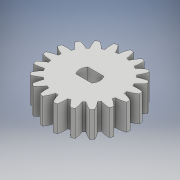
# Autodesk Inventor part: Gear19
Saved by Autodesk Inventor 2018.3 (Build 223284000, 284)
## iProperties
Created: 2019-04-15
Part Number: Gear19
Material: 一般
Document SubType Name: Modeling
Designer: shun2
Density: 1 g/cm^3
Appearance: 既定
Author: shun2
Autodesk Inventor part; units mm, degrees
ref_plane "YZ Plane" through (0, 0, 0) normal (1, 0, 0) x (0, 1, 0)
ref_plane "XZ Plane" through (0, 0, 0) normal (0, 1, 0) x (-1, 0, 0)
ref_plane "XY Plane" through (0, 0, 0) normal (0, 0, 1) x (1, 0, 0)
sketch "スケッチ1" plane through (0, 0, 0) normal (0, 0, 1) x (1, 0, 0)
  arc A0 (-3.8168, 9.7817) -> (-3.6234, 7.4117) centre (4.2362, 9.2462) ccw
  arc A1 (-3.6234, 7.4117) -> (-4.2231, 7.0872) centre (0, 0) ccw
  arc A2 (-4.2231, 7.0872) -> (-6.1013, 8.5454) centre (-10.0576, 1.5108) ccw
  arc A3 (-6.1013, 8.5454) -> (-6.7861, 8.0124) centre (0, 0) ccw
  arc A4 (-6.7861, 8.0124) -> (-5.8336, 5.8336) centre (1.0044, 10.1207) ccw
  arc A5 (-5.8336, 5.8336) -> (-6.2954, 5.332) centre (0, 0) ccw
  arc A6 (-6.2954, 5.332) -> (-8.5454, 6.1013) centre (-10.0032, -1.8368) ccw
  arc A7 (-8.5454, 6.1013) -> (-9.0201, 5.3748) centre (0, 0) ccw
  arc A8 (-9.0201, 5.3748) -> (-7.4117, 3.6234) centre (-2.3362, 9.8985) ccw
  arc A9 (-7.4117, 3.6234) -> (-7.6856, 2.9989) centre (0, 0) ccw
  arc A10 (-7.6856, 2.9989) -> (-10.0635, 2.996) centre (-8.8648, -4.9853) ccw
  arc A11 (-10.0635, 2.996) -> (-10.2765, 2.1548) centre (0, 0) ccw
  arc A12 (-10.2765, 2.1548) -> (-8.1866, 1.0205) centre (-5.4236, 8.6036) ccw
  arc A13 (-8.1866, 1.0205) -> (-8.243, 0.3409) centre (0, 0) ccw
  arc A14 (-8.243, 0.3409) -> (-10.491, -0.4339) centre (-6.7658, -7.5935) ccw
  arc A15 (-10.491, -0.4339) -> (-10.4194, -1.2988) centre (0, 0) ccw
  arc A16 (-10.4194, -1.2988) -> (-8.0744, -1.693) centre (-7.9233, 6.3764) ccw
  arc A17 (-8.0744, -1.693) -> (-7.907, -2.354) centre (0, 0) ccw
  arc A18 (-7.907, -2.354) -> (-9.7817, -3.8168) centre (-3.9336, -9.3789) ccw
  arc A19 (-9.7817, -3.8168) -> (-9.4331, -4.6116) centre (0, 0) ccw
  arc A20 (-9.4331, -4.6116) -> (-7.0872, -4.2231) centre (-9.5644, 3.4582) ccw
  arc A21 (-7.0872, -4.2231) -> (-6.7143, -4.7939) centre (0, 0) ccw
  arc A22 (-6.7143, -4.7939) -> (-8.0124, -6.7861) centre (-0.6751, -10.148) ccw
  arc A23 (-8.0124, -6.7861) -> (-7.4246, -7.4246) centre (0, 0) ccw
  arc A24 (-7.4246, -7.4246) -> (-5.332, -6.2954) centre (-10.1691, 0.1652) ccw
  arc A25 (-5.332, -6.2954) -> (-4.7939, -6.7143) centre (0, 0) ccw
  arc A26 (-4.7939, -6.7143) -> (-5.3748, -9.0201) centre (2.6565, -9.8173) ccw
  arc A27 (-5.3748, -9.0201) -> (-4.6116, -9.4331) centre (0, 0) ccw
  arc A28 (-4.6116, -9.4331) -> (-2.9989, -7.6856) centre (-9.6717, -3.1456) ccw
  arc A29 (-2.9989, -7.6856) -> (-2.354, -7.907) centre (0, 0) ccw
  arc A30 (-2.354, -7.907) -> (-2.1548, -10.2765) centre (5.7003, -8.4228) ccw
  arc A31 (-2.1548, -10.2765) -> (-1.2988, -10.4194) centre (0, 0) ccw
  arc A32 (-1.2988, -10.4194) -> (-0.3409, -8.243) centre (-8.1263, -6.1156) ccw
  arc A33 (-0.3409, -8.243) -> (0.3409, -8.243) centre (0, 0) ccw
  arc A34 (0.3409, -8.243) -> (1.2988, -10.4194) centre (8.1263, -6.1156) ccw
  arc A35 (1.2988, -10.4194) -> (2.1548, -10.2765) centre (0, 0) ccw
  arc A36 (2.1548, -10.2765) -> (2.354, -7.907) centre (-5.7003, -8.4228) ccw
  arc A37 (2.354, -7.907) -> (2.9989, -7.6856) centre (0, 0) ccw
  arc A38 (2.9989, -7.6856) -> (4.6116, -9.4331) centre (9.6717, -3.1456) ccw
  arc A39 (4.6116, -9.4331) -> (5.3748, -9.0201) centre (0, 0) ccw
  arc A40 (5.3748, -9.0201) -> (4.7939, -6.7143) centre (-2.6565, -9.8173) ccw
  arc A41 (4.7939, -6.7143) -> (5.332, -6.2954) centre (0, 0) ccw
  arc A42 (5.332, -6.2954) -> (7.4246, -7.4246) centre (10.1691, 0.1652) ccw
  arc A43 (7.4246, -7.4246) -> (8.0124, -6.7861) centre (0, 0) ccw
  arc A44 (8.0124, -6.7861) -> (6.7143, -4.7939) centre (0.6751, -10.148) ccw
  arc A45 (6.7143, -4.7939) -> (7.0872, -4.2231) centre (0, 0) ccw
  arc A46 (7.0872, -4.2231) -> (9.4331, -4.6116) centre (9.5644, 3.4582) ccw
  arc A47 (9.4331, -4.6116) -> (9.7817, -3.8168) centre (0, 0) ccw
  arc A48 (9.7817, -3.8168) -> (7.907, -2.354) centre (3.9336, -9.3789) ccw
  arc A49 (7.907, -2.354) -> (8.0744, -1.693) centre (0, 0) ccw
  arc A50 (8.0744, -1.693) -> (10.4194, -1.2988) centre (7.9233, 6.3764) ccw
  arc A51 (10.4194, -1.2988) -> (10.491, -0.4339) centre (0, 0) ccw
  arc A52 (10.491, -0.4339) -> (8.243, 0.3409) centre (6.7658, -7.5935) ccw
  arc A53 (8.243, 0.3409) -> (8.1866, 1.0205) centre (0, 0) ccw
  arc A54 (8.1866, 1.0205) -> (10.2765, 2.1548) centre (5.4236, 8.6036) ccw
  arc A55 (10.2765, 2.1548) -> (10.0635, 2.996) centre (0, 0) ccw
  arc A56 (10.0635, 2.996) -> (7.6856, 2.9989) centre (8.8648, -4.9853) ccw
  arc A57 (7.6856, 2.9989) -> (7.4117, 3.6234) centre (0, 0) ccw
  arc A58 (7.4117, 3.6234) -> (9.0201, 5.3748) centre (2.3362, 9.8985) ccw
  arc A59 (9.0201, 5.3748) -> (8.5454, 6.1013) centre (0, 0) ccw
  arc A60 (8.5454, 6.1013) -> (6.2954, 5.332) centre (10.0032, -1.8368) ccw
  arc A61 (6.2954, 5.332) -> (5.8336, 5.8336) centre (0, 0) ccw
  arc A62 (5.8336, 5.8336) -> (6.7861, 8.0124) centre (-1.0044, 10.1207) ccw
  arc A63 (6.7861, 8.0124) -> (6.1013, 8.5454) centre (0, 0) ccw
  arc A64 (6.1013, 8.5454) -> (4.2231, 7.0872) centre (10.0576, 1.5108) ccw
  arc A65 (4.2231, 7.0872) -> (3.6234, 7.4117) centre (0, 0) ccw
  arc A66 (3.6234, 7.4117) -> (3.8168, 9.7817) centre (-4.2362, 9.2462) ccw
  arc A67 (3.8168, 9.7817) -> (2.996, 10.0635) centre (0, 0) ccw
  arc A68 (2.996, 10.0635) -> (1.693, 8.0744) centre (9.0221, 4.6946) ccw
  arc A69 (1.693, 8.0744) -> (1.0205, 8.1866) centre (0, 0) ccw
  arc A70 (1.0205, 8.1866) -> (0.4339, 10.491) centre (-7.0089, 7.3697) ccw
  arc A71 (0.4339, 10.491) -> (-0.4339, 10.491) centre (0, 0) ccw
  arc A72 (-0.4339, 10.491) -> (-1.0205, 8.1866) centre (7.0089, 7.3697) ccw
  arc A73 (-1.0205, 8.1866) -> (-1.693, 8.0744) centre (0, 0) ccw
  arc A74 (-1.693, 8.0744) -> (-2.996, 10.0635) centre (-9.0221, 4.6946) ccw
  arc A75 (-2.996, 10.0635) -> (-3.8168, 9.7817) centre (0, 0) ccw
  line L0 (-2, 1.5) -> (2, 1.5)
  line L1 (2, -1.5) -> (-2, -1.5)
  arc A76 (2, -1.5) -> (2, 1.5) centre (0, 0) ccw
  arc A77 (-2, 1.5) -> (-2, -1.5) centre (0, 0) ccw
  point P0 (0, 0)
  point P1 (0, 0)
  point P2 (0, 0)
  point P3 (0, 0)
  point P4 (0, 0)
  point P5 (0, 0)
  point P6 (0, 0)
  point P7 (0, 0)
  point P8 (0, 0)
  point P9 (0, 0)
  point P10 (0, 0)
  point P11 (0, 0)
  point P12 (0, 0)
  point P13 (0, 0)
  point P14 (0, 0)
  point P15 (0, 0)
  point P16 (0, 0)
  point P17 (0, 0)
  point P18 (0, 0)
  point P19 (0, 0)
  point P20 (0, 0)
  point P21 (0, 0)
  point P22 (0, 0)
  point P23 (0, 0)
  point P24 (0, 0)
  point P25 (0, 0)
  point P26 (0, 0)
  point P27 (0, 0)
  point P28 (0, 0)
  point P29 (0, 0)
  point P30 (0, 0)
  point P31 (0, 0)
  point P32 (0, 0)
  point P33 (0, 0)
  point P34 (0, 0)
  constraints: 156 point on circle, 78 centre point, 4 end point, 1 coincident, 1 horizontal, 1 parallel
extrude "押し出し1" add sketch "スケッチ1" along normal blind 6.5
